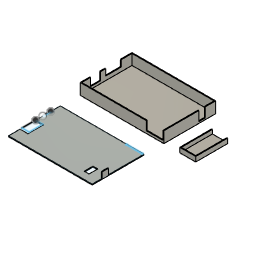
FPLock_Case (Autodesk Fusion 360 design; units mm, degrees)
Autodesk Fusion 360 part; units mm, degrees
sketch "草图1" plane through (0, 0, 0) normal (0, 1, 0) x (1, 0, 0)
  line L0 (0, 0) -> (105, 0)
  line L1 (105, 0) -> (105, 65)
  line L2 (105, 65) -> (0, 65)
  line L3 (0, 65) -> (0, 0)
  constraint horizontal L0
  constraint vertical L1
  constraint horizontal L2
  constraint vertical L3
  constraint coincident L0.start L3.end
extrude "拉伸1" add sketch "草图1" along normal blind 1 makes body 1
sketch "草图2" plane through (0, 1, 0) normal (0, 1, 0) x (-1, 0, 0)
  line L0 (0, -65) -> (0, 0)
  line L1 (0, 0) -> (-105, 0)
  line L2 (-105, 0) -> (-105, -65)
  line L3 (-105, -65) -> (0, -65)
  line L4 (-1, -1) -> (-104, -1)
  line L5 (-104, -1) -> (-104, -64)
  line L6 (-104, -64) -> (-1, -64)
  line L7 (-1, -64) -> (-1, -1)
  constraint horizontal L4
  constraint vertical L5
  constraint horizontal L6
  constraint vertical L7
extrude "拉伸2" add sketch "草图2" along normal blind 13 bodies 1
sketch "草图3" plane through (0, 0, 0) normal (0, 0, 1) x (1, 0, 0)
  line L0 (0, 0) -> (105, 0)
  line L1 (105, 0) -> (105, 14)
  line L2 (105, 14) -> (0, 14)
  line L3 (0, 14) -> (0, 0)
  line L4 (104, 1) -> (83, 1)
  line L5 (83, 1) -> (83, 14)
  line L6 (83, 14) -> (104, 14)
  line L7 (104, 14) -> (104, 1)
  dimension "d5" = 21
  constraint horizontal L4
  constraint vertical L5
  constraint horizontal L6
  constraint vertical L7
  measures "d5" distance of L4.start L4.end
extrude "拉伸3" cut sketch "草图3" against normal blind 1 contours L2 L4 L5 L6 L7 bodies 1
sketch "草图4" plane through (0, 0, 0) normal (-1, 0, 0) x (0, 0, 1)
  line L0 (-65, 0) -> (0, 0)
  line L1 (0, 0) -> (0, 14)
  line L2 (0, 14) -> (-65, 14)
  line L3 (-65, 14) -> (-65, 0)
  line L4 (-12, 6) -> (-22, 6)
  line L5 (-22, 6) -> (-22, 11)
  line L6 (-22, 11) -> (-12, 11)
  line L7 (-12, 11) -> (-12, 6)
  line L8 (-22, 11) -> (-12, 11)
  line L9 (-12, 11) -> (-12, 14)
  line L10 (-12, 14) -> (-22, 14)
  line L11 (-22, 14) -> (-22, 11)
  line L12 (-31, 6) -> (-48, 6)
  line L13 (-48, 6) -> (-48, 14)
  line L14 (-48, 14) -> (-31, 14)
  line L15 (-31, 14) -> (-31, 6)
  constraint horizontal L4
  constraint vertical L5
  constraint horizontal L6
  constraint vertical L7
  constraint horizontal L8
  constraint vertical L9
  constraint horizontal L10
  constraint vertical L11
  constraint coincident L2 L9.end
  constraint horizontal L12
  constraint vertical L13
  constraint horizontal L14
  constraint vertical L15
  constraint coincident L2 L13.end
extrude "拉伸4" cut sketch "草图4" against normal blind 1 contours L2 L12 L13 L14 L15 | L2 L6 L8 L9 L10 L11 | L4 L5 L6 L7 L8 bodies 1
sketch "草图5" plane through (0, 0, 0) normal (0, 1, 0) x (1, 0, 0)
  line L0 (0, -25) -> (105, -25)
  line L1 (105, -25) -> (105, -90)
  line L2 (105, -90) -> (0, -90)
  line L3 (0, -90) -> (0, -25)
  constraint horizontal L0
  constraint vertical L1
  constraint horizontal L2
  constraint vertical L3
extrude "拉伸5" add sketch "草图5" along normal blind 1 separate body makes body 2
sketch "草图6" plane through (0, 1, 0) normal (0, 1, 0) x (-1, 0, 0)
  line L0 (0, 90) -> (-105, 90)
  line L1 (-105, 90) -> (-105, 25)
  line L2 (-105, 25) -> (0, 25)
  line L3 (0, 25) -> (0, 90)
  line L4 (-103.5, 26) -> (-83.5, 26)
  line L5 (-83.5, 26) -> (-83.5, 25)
  line L6 (-83.5, 25) -> (-103.5, 25)
  line L7 (-103.5, 25) -> (-103.5, 26)
  line L8 (0, 47) -> (0, 37)
  line L9 (-1, 46.5) -> (0, 46.5)
  line L10 (0, 46.5) -> (0, 37.5)
  line L11 (0, 37.5) -> (-1, 37.5)
  line L12 (-1, 37.5) -> (-1, 46.5)
  line L13 (0, 56) -> (-9, 56)
  line L14 (-9, 56) -> (-9, 73)
  line L15 (-9, 73) -> (0, 73)
  line L16 (0, 73) -> (0, 56)
  dimension "d13" = 20
  constraint horizontal L4
  constraint vertical L5
  constraint horizontal L6
  constraint vertical L7
  constraint vertical L8
  constraint coincident L3 L8.end
  constraint horizontal L9
  constraint vertical L10
  constraint horizontal L11
  constraint vertical L12
  constraint coincident L8 L10.end
  constraint horizontal L13
  constraint vertical L14
  constraint horizontal L15
  constraint vertical L16
  constraint coincident L3 L13.start
  measures "d13" distance of L4.start L4.end
extrude "拉伸7" cut sketch "草图6" against normal blind 1 contours L3 L13 L14 L15 L16 bodies 2
extrude "拉伸8" add sketch "草图6" along normal blind 2 contours L3 L8 L9 L10 L11 L12 bodies 2
sketch "草图7" plane through (0, 14, 0) normal (0, 1, 0) x (-1, 0, 0)
  line L0 (0, -48) -> (-1, -48)
  line L1 (-1, -48) -> (-1, -64)
  line L2 (-1, -64) -> (-104, -64)
  line L3 (-104, -64) -> (-104, 0)
  line L4 (-104, 0) -> (-105, 0)
  line L5 (-105, 0) -> (-105, -65)
  line L6 (-105, -65) -> (0, -65)
  line L7 (0, -65) -> (0, -48)
  line L8 (-105, -52) -> (-104, -52)
  line L9 (-104, -52) -> (-104, -44)
  line L10 (-104, -44) -> (-105, -44)
  line L11 (-105, -44) -> (-105, -52)
  constraint horizontal L8
  constraint vertical L9
  constraint horizontal L10
  constraint vertical L11
  constraint coincident L3 L9.end
  constraint coincident L5 L8.start
extrude "拉伸9" cut sketch "草图7" against normal blind 12 contours L3 L5 L8 L9 L10 L11 bodies 1
sketch "草图8" plane through (0, 1, 0) normal (0, 1, 0) x (-1, 0, 0)
  line L0 (-105, 77.5) -> (-104, 77.5)
  line L1 (-104, 77.5) -> (-104, 69.5)
  line L2 (-104, 69.5) -> (-105, 69.5)
  line L3 (-105, 69.5) -> (-105, 77.5)
  constraint horizontal L0
  constraint vertical L1
  constraint horizontal L2
  constraint vertical L3
extrude "拉伸10" add sketch "草图8" along normal blind 7 bodies 2
sketch "草图9" plane through (0, 1, 0) normal (0, 1, 0) x (-1, 0, 0)
  line L0 (-94, 83) -> (-89, 83)
  line L1 (-89, 83) -> (-89, 73)
  line L2 (-89, 73) -> (-94, 73)
  line L3 (-94, 73) -> (-94, 83)
  constraint horizontal L0
  constraint vertical L1
  constraint horizontal L2
  constraint vertical L3
sketch "草图10" plane through (0, 0, 0) normal (0, 1, 0) x (1, 0, 0)
  line L0 (125, 0) -> (145, 0)
  line L1 (145, 0) -> (145, 40)
  line L2 (145, 40) -> (125, 40)
  line L3 (125, 40) -> (125, 0)
  constraint horizontal L0
  constraint vertical L1
  constraint horizontal L2
  constraint vertical L3
extrude "拉伸12" add sketch "草图10" along normal blind 1 separate body makes body 3
sketch "草图11" plane through (0, 1, 0) normal (0, 1, 0) x (-1, 0, 0)
  line L0 (-125, -40) -> (-125, 0)
  line L1 (-125, 0) -> (-145, 0)
  line L2 (-145, 0) -> (-145, -40)
  line L3 (-145, -40) -> (-125, -40)
  line L4 (-144, -1) -> (-126, -1)
  line L5 (-126, -1) -> (-126, -40)
  line L6 (-126, -40) -> (-144, -40)
  line L7 (-144, -40) -> (-144, -1)
  dimension "d28" = 18
  constraint horizontal L4
  constraint vertical L5
  constraint horizontal L6
  constraint vertical L7
  measures "d28" distance of L4.start L4.end
extrude "拉伸13" add sketch "草图11" along normal blind 5 contours L0 L1 L2 L3 L4 L5 L7 bodies 3
sketch "草图12" plane through (0, 1, 0) normal (0, 1, 0) x (-1, 0, 0)
  line L0 (-1, -1) -> (-83, -1)
  line L1 (-83, -1) -> (-83, 0)
  line L2 (-83, 0) -> (-104, 0)
  line L3 (-104, 0) -> (-104, -64)
  line L4 (-104, -64) -> (-1, -64)
  line L5 (-1, -64) -> (-1, -1)
  line L6 (-83, -1) -> (-104, -1)
  line L7 (-104, -1) -> (-104, 0)
  line L8 (-104, 0) -> (-83, 0)
  line L9 (-83, 0) -> (-83, -1)
  constraint horizontal L6
  constraint vertical L7
  constraint horizontal L8
  constraint vertical L9
  constraint coincident L2.end L3.start
  constraint coincident L0.end L1.start
extrude "拉伸14" add sketch "草图12" along normal blind 2 contours L1 L2 L3 L6 L7 L8 L9 bodies 1
sketch "草图13" plane through (0, 1, 0) normal (0, 1, 0) x (-1, 0, 0)
  line L0 (-86, 70) -> (-92, 70)
  line L1 (-92, 70) -> (-92, 81)
  line L2 (-92, 81) -> (-86, 81)
  line L3 (-86, 81) -> (-86, 70)
  constraint horizontal L0
  constraint vertical L1
  constraint horizontal L2
  constraint vertical L3
extrude "拉伸15" cut sketch "草图13" against normal blind 1 bodies 2
extrude "拉伸16" cut 1 faces at (0.3333, 8.6667, -48) along direction (0, 0, -1) blind 2.5 on bodies 1 bodies 1
extrude "拉伸17" cut 1 faces at (0.3333, 11.3333, -22) along direction (0, 0, -1) blind 2.5 on bodies 1 bodies 1
extrude "拉伸18" cut 1 faces at (0.3333, 6, -16.1667) along direction (0, -1, 0) blind 2 on bodies 1 bodies 1
extrude "拉伸19" add 1 faces at (0.6667, 1.6667, 46.5) along direction (0, 0, 1) blind 2.5 on bodies 2 bodies 2
extrude "拉伸20" cut 1 faces at (6, 0.6667, 73) along direction (0, 0, 1) blind 2.5 on bodies 2 bodies 2
extrude "拉伸21" cut 1 faces at (9, 0.3333, 69) along direction (1, 0, 0) blind 1 on bodies 2 bodies 2
extrude "拉伸22" cut 1 faces at (0.3333, 3, 45.1667) along direction (0, -1, 0) blind 2 on bodies 2 bodies 2
